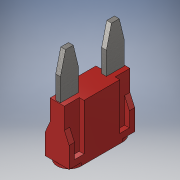
# Autodesk Inventor part: Mini car fuse
Saved by Autodesk Inventor 2019 (Build 230136000, 136)
## iProperties
Created: 2019-08-23
Part Number: Mini car fuse
Material: Generic
Document SubType Name: Modeling
Designer: Andras
Density: 1 g/cm^3
Appearance: Default
Author: Andras
Autodesk Inventor part; units mm, degrees
ref_plane "YZ Plane" through (0, 0, 0) normal (1, 0, 0) x (0, 1, 0)
sketch "Sketch1" plane through (0, 0, 0) normal (0, 1, 0) x (-1, 0, 0)
  line L0 (0, 0) -> (4, 0)
  line L1 (4, 0) -> (4, -11)
  line L2 (4, -11) -> (0, -11)
  line L3 (0, -11) -> (0, 0)
  dimension "d0" = 4
  dimension "d1" = 11
  constraints: 8 end point, 2 parallel, 1 horizontal, 1 perpendicular
  measures "d0" distance of L1.end L2.end
  measures "d1" distance of L0.end L1.end
extrude "Extrusion1" add sketch "Sketch1" along normal blind 9.3
sketch "Sketch2" plane through (0, 9.3, 0) normal (0, 1, 0) x (1, 0, 0)
  line L0 (-4, 0) -> (0, 0) projected
  line L1 (0, 0) -> (0, 11) projected
  line L2 (0, 11) -> (-4, 11) construction
  line L3 (-4, 11) -> (-4, 0) projected
  line L4 (0, 11) -> (-4, 11) construction
  line L5 (-2.4, 0.15) -> (-1.6, 0.15)
  line L6 (-1.6, 0.15) -> (-1.6, 10.85)
  line L7 (-1.6, 10.85) -> (-2.4, 10.85)
  line L8 (-2.4, 10.85) -> (-2.4, 0.15)
  dimension "d5" = 0.8
  dimension "d6" = 4
  dimension "d7" = 1.6
  dimension "d40" = 0.15
  dimension "d41" = 0.15
  constraints: 8 end point, 1 horizontal, 1 parallel, 1 perpendicular
  measures "d5" distance between parallel lines of L6 L8
  measures "d6" distance of L1.end L2.end
  measures "d7" distance between parallel lines of L8 L3
  measures "d40" distance between parallel lines of L0 L5
  measures "d41" distance between parallel lines of L2 L7
extrude "Extrusion2" add sketch "Sketch2" along normal blind 7.3
sketch "Sketch3" plane through (-1.6, 9.3, -0.15) normal (1, 0, 0) x (0, 0, -1)
  line L0 (10.7, 0) -> (0, 0) projected
  line L1 (10.7, 0) -> (10.7, 7.3) projected
  line L2 (0, 7.3) -> (10.7, 7.3) projected
  line L3 (0, 0) -> (0, 7.3) projected
  line L4 (0, 7.3) -> (10.7, 7.3) projected
  line L5 (0, 0) -> (10.7, 0) projected
  line L6 (3, 7.3) -> (7.7, 7.3)
  line L7 (7.7, 7.3) -> (7.7, 0)
  line L8 (7.7, 0) -> (3, 0)
  line L9 (3, 0) -> (3, 7.3)
  point P0 (-0.15, -9.3)
  dimension "d10" = 3
  dimension "d11" = 3
  constraints: 8 end point, 2 parallel, 2 point on line, 1 horizontal, 1 perpendicular
  measures "d10" distance between parallel lines of L1 L7
  measures "d11" distance between parallel lines of L3 L9
extrude "Extrusion3" cut sketch "Sketch3" against normal blind 9.3 contours L0 L9 L2 L7
chamfer "Chamfer1" distance 0.85 distance2 3.5 1 edges at (-2, 16.6, -3.15) measured on face at (-2.1333, 16.6, -2.15)
chamfer "Chamfer2" distance 0.85 distance2 3.5 1 edges at (-2, 16.6, -0.15) measured on face at (-2.1333, 16.6, -1.5833)
chamfer "Chamfer3" distance 0.85 distance2 3.5 1 edges at (-2, 16.6, -7.85) measured on face at (-2.1333, 16.6, -9.85)
chamfer "Chamfer4" distance 0.85 distance2 3.5 1 edges at (-2, 16.6, -10.85) measured on face at (-2.1333, 16.6, -10.1333)
sketch "Sketch4" plane through (0, 0, 0) normal (0, -1, 0) x (1, 0, 0)
  line L0 (0, 0) -> (-4, 0) projected
  line L1 (-4, 0) -> (-4, -11) projected
  line L2 (-4, -11) -> (0, -11) projected
  line L3 (0, -11) -> (0, 0) projected
  line L4 (-2, -2) -> (-2, -9) construction
  line L5 (-4, -2) -> (-4, -9)
  line L6 (0, -9) -> (0, -2)
  arc A0 (0, -2) -> (-4, -2) centre (-2, -2) ccw
  arc A1 (-4, -9) -> (0, -9) centre (-2, -9) ccw
  line L7 (0, 0) -> (-4, 0) projected
  line L8 (0, -11) -> (0, 0) projected
  point P0 (-2, -5.5)
  constraints: 8 end point, 8 tangent, 4 point on circle, 2 centre point, 1 midpoint, 1 parallel, 1 vertical
extrude "Extrusion4" cut sketch "Sketch4" against normal blind 0.5 contours L3 A0 L0 | A0 L1 L0 | L3 L2 A1 | A1 L2 L1
sketch "Sketch5" plane through (-4, 9.3, -11) normal (-1, 0, 0) x (0, 0, 1)
  line L0 (0, -8.8) -> (2, -8.8) projected
  line L1 (2, -8.8) -> (2, -9.3) projected
  line L2 (9, -9.3) -> (2, -9.3) construction
  line L3 (9, -8.8) -> (9, -9.3) projected
  line L4 (9, -8.8) -> (11, -8.8) projected
  line L5 (11, -8.8) -> (11, 0) projected
  line L6 (0, 0) -> (11, 0) projected
  line L7 (0, -8.8) -> (0, 0) projected
  line L8 (10.1, 0) -> (8.5, 0)
  line L9 (8.5, 0) -> (8.5, -7.8)
  line L10 (8.5, -7.8) -> (10.1, -7.8)
  line L11 (10.1, -7.8) -> (10.1, 0)
  line L12 (11, 0) -> (0, 0) projected
  line L13 (0.9, 0) -> (2.5, 0)
  line L14 (2.5, 0) -> (2.5, -7.8)
  line L15 (2.5, -7.8) -> (0.9, -7.8)
  line L16 (0.9, -7.8) -> (0.9, 0)
  point P0 (11, -9.3)
  dimension "d28" = 0.9
  dimension "d29" = 0.9
  dimension "d30" = 1.6
  dimension "d31" = 1.6
  dimension "d32" = 1.5
  constraints: 16 end point, 4 parallel, 3 point on line, 2 horizontal, 2 perpendicular
  measures "d28" distance between parallel lines of L7 L16
  measures "d29" distance between parallel lines of L5 L11
  measures "d30" distance of L9.end L10.end
  measures "d31" distance between parallel lines of L16 L14
  measures "d32" distance between parallel lines of L15 L2
extrude "Extrusion5" cut sketch "Sketch5" against normal blind 0.8
ref_plane "Work Plane1" through (-2, 0, -9) normal (-1, 0, 0) x (0, 0, 1)
mirror "Mirror1" about plane through (-2, 0, -9) normal (-1, 0, 0) of "Extrusion5"
sketch "Sketch6" plane through (-1.6, 9.3, 0) normal (0, 0, 1) x (1, 0, 0)
  line L0 (0.8, 0) -> (0.8, -7.8) projected
  line L1 (0.8, -7.8) -> (0.8, 0) projected
  line L2 (-1.6, -7.8) -> (-1.6, 0) projected
  line L3 (0.8, 0) -> (0.8, -7.8) projected
  line L4 (0.8, -3.5) -> (1.6, -5.3)
  line L5 (1.6, 0) -> (1.6, -7.8) projected
  line L6 (-2.4, -9.3) -> (1.6, -9.3) projected
  line L7 (0.8, 0) -> (1.6, 0) projected
  line L8 (0.8, 0) -> (1.6, 0)
  dimension "d36" = 3.5
  dimension "d37" = 4
  constraints: 4 end point, 2 point on line, 1 horizontal
  measures "d36" distance of L1.end L4.start
  measures "d37" distance from line of L6 L4.end
extrude "Extrusion6" cut sketch "Sketch6" against normal blind 1.2
mirror "Mirror2" about plane through (-2, 0, -9) normal (-1, 0, 0) of "Extrusion6"
ref_plane "Work Plane2" through (-2.4, 12.4824, -5.5) normal (0, 0, 1) x (1, 0, 0)
mirror "Mirror3" about plane through (-2.4, 12.4824, -5.5) normal (0, 0, 1) of "Extrusion6", "Mirror2"
equation "\"d7\" = -0.5 * d5 + 0.5 * d6"
equation "\"d31\" = d30"
body "Solid1"
